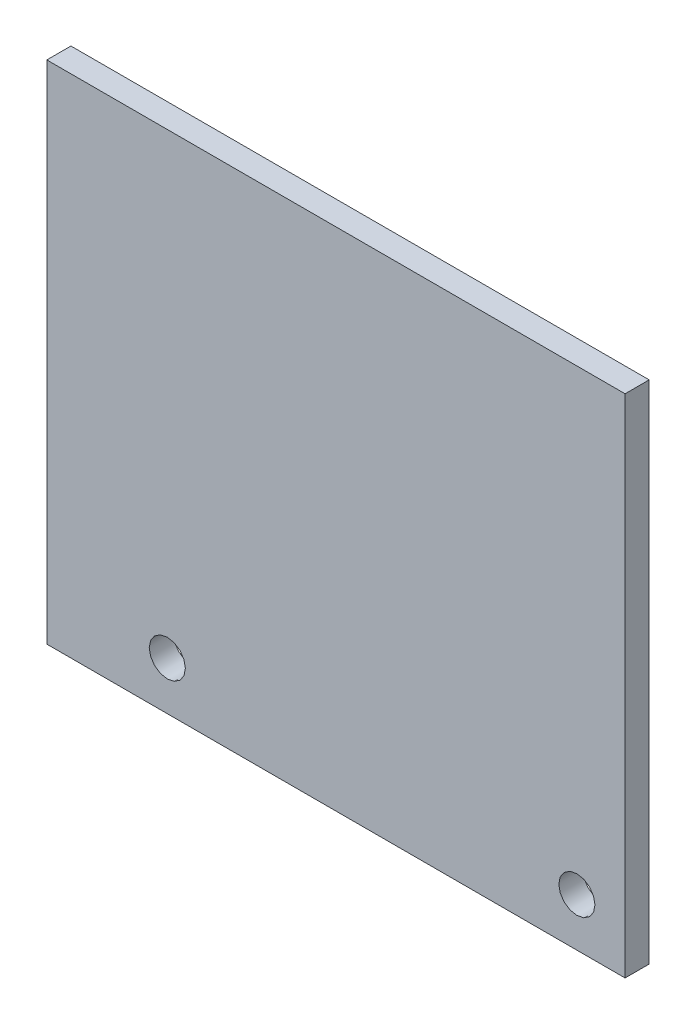
# Autodesk Inventor part: driver kort
Saved by Autodesk Inventor 2015 (Build 190159000, 159)
## iProperties
Created: 2015-08-04
Part Number: driver kort
Material: Generic
Document SubType Name: Modeling
Designer: Simen
Density: 1 g/cm^3
Appearance: Default
Author: Simen
Autodesk Inventor part; units mm, degrees
ref_plane "YZ Plane" through (0, 0, 0) normal (1, 0, 0) x (0, 1, 0)
ref_plane "XZ Plane" through (0, 0, 0) normal (0, 1, 0) x (-1, 0, 0)
ref_plane "XY Plane" through (0, 0, 0) normal (0, 0, 1) x (1, 0, 0)
sketch "Sketch2" plane through (0, 0, 0) normal (0, 0, 1) x (1, 0, 0)
  line L0 (-22.1612, -7.9741) -> (-70.1612, -7.9741)
  line L1 (-70.1612, -7.9741) -> (-70.1612, 34.0259)
  line L2 (-70.1612, 34.0259) -> (-22.1612, 34.0259)
  line L3 (-22.1612, 34.0259) -> (-22.1612, -7.9741)
  line L4 (-70.1612, -7.9741) -> (-70.1612, -3.9741)
  line L5 (-70.1612, -3.9741) -> (-60.1612, -3.9741)
  line L6 (-22.1612, -7.9741) -> (-22.1612, -3.9741)
  line L7 (-22.1612, -3.9741) -> (-26.1612, -3.9741)
  circle A0 centre (-60.1612, -3.9741) radius 1.5
  circle A1 centre (-26.1612, -3.9741) radius 1.5
  point P0 (0, 0)
  dimension "d0" = 48
  dimension "d1" = 42
  dimension "d2" = 4
  dimension "d3" = 10
  dimension "d4" = 4
  dimension "d5" = 4
  dimension "d6" = 3
  dimension "d7" = 3
  constraints: 16 end point, 3 perpendicular, 2 centre point, 2 coincident, 2 parallel, 2 point on line, 1 horizontal
  measures "d0" distance of L1.end L2.end
  measures "d1" distance of L0.end L1.end
  measures "d2" distance of L0.end L4.end
  measures "d3" distance of L4.end L5.end
  measures "d4" distance of L0.start L6.end
  measures "d5" distance of L6.end L7.end
  measures "d6" diameter of A0
  measures "d7" diameter of A1
extrude "Extrusion1" add sketch "Sketch2" along normal blind 2
body "Solid1"
